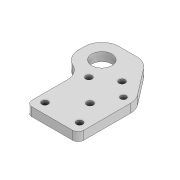
# Autodesk Inventor part: Hinge_p1_plate
Saved by Autodesk Inventor 2022 (Build 260153000, 153)
## iProperties
Created: 2022-07-11
Part Number: Hinge_p1_plate
Material: Generic
Document SubType Name: Modeling
Designer: dell
Density: 1 g/cm^3
Appearance: Default
Author: dell
Autodesk Inventor part; units mm, degrees
ref_plane "YZ Plane" through (0, 0, 0) normal (1, 0, 0) x (0, 1, 0)
ref_plane "XZ Plane" through (0, 0, 0) normal (0, 1, 0) x (-1, 0, 0)
ref_plane "XY Plane" through (0, 0, 0) normal (0, 0, 1) x (1, 0, 0)
sketch "Sketch1" plane through (0, 0, 0) normal (0, 1, 0) x (-1, 0, 0)
  line L0 (0, 0) -> (18, 0)
  line L1 (18, 0) -> (18, -18.2)
  line L2 (18, -18.2) -> (0, -18.2)
  line L3 (0, -18.2) -> (0, 0)
  line L4 (18, 0) -> (0, 0)
  line L5 (0, 0) -> (0, 2)
  line L6 (0, 2) -> (18, 2)
  line L7 (18, 2) -> (18, 0)
  circle A0 centre (3, -1.5) radius 1.1
  circle A1 centre (3, -16.7) radius 1
  circle A2 centre (15, -1.5) radius 1.1
  circle A3 centre (15, -16.7) radius 1.1
  circle A4 centre (18, -24.2) radius 3.5
  line L8 (0, -18.2) -> (25, -18.2)
  line L9 (25, -18.2) -> (25, -31.2)
  line L10 (25, -31.2) -> (0, -31.2)
  line L11 (0, -31.2) -> (0, -18.2)
  line L12 (10, -31.2) -> (0, -18.2)
  circle A5 centre (8, -21.2) radius 1.1
  dimension "d0" = 18.2
  dimension "d1" = 18
  dimension "d2" = 2
  dimension "d3" = 2.2
  dimension "d4" = 3
  dimension "d5" = 1.5
  dimension "d6" = 2
  dimension "d7" = 2.2
  dimension "d8" = 2.2
  dimension "d9" = 1.5
  dimension "d10" = 3
  dimension "d11" = 3
  dimension "d12" = 1.5
  dimension "d13" = 1.5
  dimension "d14" = 3
  dimension "d17" = 7
  dimension "d19" = 6
  dimension "d20" = 7
  dimension "d22" = 7
  dimension "d23" = 18
  dimension "d24" = 8
  dimension "d36" = 2.2
  dimension "d37" = 3
  dimension "d38" = 10
  constraints: 26 end point, 6 centre point, 6 parallel, 3 horizontal, 3 perpendicular, 3 point on line
  measures "d0" distance between parallel lines of L2 L0
  measures "d1" distance between parallel lines of L1 L3
  measures "d2" distance between parallel lines of L0 L6
  measures "d3" diameter of A0
  measures "d4" distance from line of L3 A0.centre
  measures "d5" distance from line of L0 A0.centre
  measures "d6" diameter of A1
  measures "d7" diameter of A2
  measures "d8" diameter of A3
  measures "d9" distance from line of L0 A2.centre
  measures "d10" distance from line of L1 A2.centre
  measures "d11" distance from line of L1 A3.centre
  measures "d12" distance from line of L2 A3.centre
  measures "d13" distance from line of L2 A1.centre
  measures "d14" distance from line of L3 A1.centre
  measures "d17" diameter of A4
  measures "d19" distance from line of L2 A4.centre
  measures "d20" distance between parallel lines of L1 L9
  measures "d22" distance from line of A4.centre L10
  measures "d23" distance from line of A4.centre L11
  measures "d24" horizontal distance of L12.start A4.centre
  measures "d36" diameter of A5
  measures "d37" distance from line of L8 A5.centre
  measures "d38" distance from line of L1 A5.centre
extrude "Extrusion1" add sketch "Sketch1" along normal blind 3 contours L5 L6 L7 L0 | L0 L1 L2 L3 | L2 L8 L9 L10 L12
fillet "Fillet1" radius 2 2 edges at (-18, 1.5, 2) (0, 1.5, 2)
fillet "Fillet2" radius 6 5 edges at (0, 1.5, -18.2) (-25, 1.5, -18.2) (-25, 1.5, -31.2) (-10, 1.5, -31.2) (-18, 1.5, -18.2)
sketch "Sketch3" plane through (0, 3, 0) normal (0, 1, 0) x (1, 0, 0)
  circle A0 centre (-7, 9.1) radius 1.15
  line L0 (-16, -2) -> (-2, -2) projected
  line L1 (0, 0) -> (0, 16.1593) projected
  line L2 (-18, 12.2) -> (-18, 0) projected
  point P0 (0, 16.2)
  dimension "d29" = 2.3
  dimension "d34" = 11
  dimension "d35" = 11.1
  constraints: 1 centre point
  measures "d29" diameter of A0
  measures "d34" distance from line of L2 A0.centre
  measures "d35" distance from line of L0 A0.centre
extrude "Extrusion2" cut sketch "Sketch3" along normal mid plane 100
sketch "Sketch2" plane through (0, 3, 0) normal (0, 1, 0) x (1, 0, 0)
  circle A0 centre (-18, 24.2) radius 3.5 projected
  circle A1 centre (-15, 16.7) radius 1.1 projected
  circle A2 centre (-15, 1.5) radius 1.1 projected
  circle A3 centre (-3, 16.7) radius 1 projected
  circle A4 centre (-3, 1.5) radius 1.1 projected
  arc A5 (-25, 23.1087) -> (-21.5, 17.6544) centre (-19, 23.1087) ccw projected
  arc A6 (-18, 12.2) -> (-21.5, 17.6544) centre (-24, 12.2) ccw projected
  line L0 (-18, 12.2) -> (-18, 0) projected
  arc A7 (-18, 0) -> (-16, -2) centre (-16, 0) ccw projected
  line L1 (-16, -2) -> (-2, -2) projected
  arc A8 (-2, -2) -> (0, 0) centre (-2, 0) ccw projected
  line L2 (0, 0) -> (0, 16.1593) projected
  arc A9 (0, 16.1593) -> (-1.2443, 19.8175) centre (-6, 16.1593) ccw projected
  line L3 (-1.2443, 19.8175) -> (-8.1987, 28.8583) projected
  arc A10 (-8.1987, 28.8583) -> (-12.9544, 31.2) centre (-12.9544, 25.2) ccw projected
  line L4 (-12.9544, 31.2) -> (-19, 31.2) projected
  arc A11 (-19, 31.2) -> (-25, 25.2) centre (-19, 25.2) ccw projected
  line L5 (-25, 25.2) -> (-25, 23.1087) projected
  circle A12 centre (-7, 9.1) radius 1.15 projected
  circle A13 centre (-18, 24.2) radius 3.5 projected
  circle A14 centre (-15, 16.7) radius 1.1 projected
  circle A15 centre (-15, 1.5) radius 1.1 projected
  circle A16 centre (-3, 16.7) radius 1 projected
  circle A17 centre (-3, 1.5) radius 1.1 projected
  arc A18 (-25, 23.1087) -> (-21.5, 17.6544) centre (-19, 23.1087) ccw projected
  arc A19 (-18, 12.2) -> (-21.5, 17.6544) centre (-24, 12.2) ccw projected
  line L6 (-18, 12.2) -> (-18, 0) projected
  arc A20 (-18, 0) -> (-16, -2) centre (-16, 0) ccw projected
  line L7 (-16, -2) -> (-2, -2) projected
  arc A21 (-2, -2) -> (0, 0) centre (-2, 0) ccw projected
  line L8 (0, 0) -> (0, 16.1593) projected
  arc A22 (0, 16.1593) -> (-1.2443, 19.8175) centre (-6, 16.1593) ccw projected
  line L9 (-1.2443, 19.8175) -> (-8.1987, 28.8583) projected
  arc A23 (-8.1987, 28.8583) -> (-12.9544, 31.2) centre (-12.9544, 25.2) ccw projected
  line L10 (-12.9544, 31.2) -> (-19, 31.2) projected
  arc A24 (-19, 31.2) -> (-25, 25.2) centre (-19, 25.2) ccw projected
  line L11 (-25, 25.2) -> (-25, 23.1087) projected
  point P0 (0, 0)
body "Solid1"
